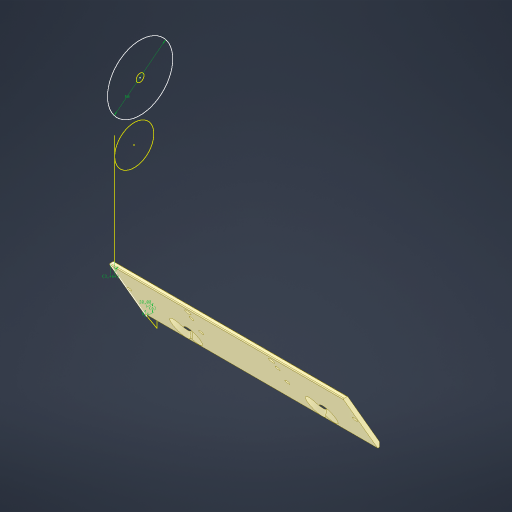
# Autodesk Inventor part: front
Saved by Autodesk Inventor 2023 (Build 270158000, 158)
## iProperties
Created: 2024-05-26
Part Number: front
Material: Nylon 6
Document SubType Name: Modeling
Designer: szymo
Density: 1.12 g/cm^3
Appearance: Nylon 6
Mass: 18.6267 g
Surface Area: 186.523 cm^2
Volume: 16.631 cm^3
TOTAL MASS: 0.0
Author: szymo
Autodesk Inventor part; units mm, degrees
ref_plane "Work Plane1" through (-178, 0.5, -3.5) normal (-1, 0, 0) x (0, 0, 1)
sketch "Sketch1" plane through (-178, 0.5, -3.5) normal (-1, 0, 0) x (0, 0, 1)
  line L0 (3.5, 3.5) -> (-1, 3.5) projected
  line L1 (-1, 3.5) -> (-1, -0.5) projected
  line L2 (-1, -0.5) -> (-4.5, -0.5) projected
  line L3 (-4.5, -0.5) -> (-4.5, -14.5) projected
  line L4 (-4.5, -14.5) -> (4.5, -0.5) projected
  line L5 (4.5, -0.5) -> (3.5, -0.5) projected
  line L6 (3.5, -0.5) -> (3.5, 3.5) projected
  circle A0 centre (8.5, 158.5) radius 3 projected
  circle A1 centre (8.5, 158.5) radius 25
  circle A2 centre (13, 116) radius 15 projected
  line L7 (3.5, 3.5) -> (28, 45.9352)
  line L8 (3.5, -2.5) -> (31.4641, 45.9352)
  line L9 (31.4641, 45.9352) -> (28, 45.9352)
  line L10 (28, 45.9352) -> (28, 130) projected
  line L11 (3.5, -2.5) -> (3.5, -0.5)
  line L12 (3.5, -0.1) -> (4.8856, -0.1)
  point P0 (4.0774, -0.5)
  point P1 (3.5, -2.0556)
  dimension "d0" = 50
  dimension "d1" = 30
  dimension "d3" = 3
  dimension "d4" = 6
  dimension "d5" = 3.4641
  dimension "d49" = 0.4
  constraints: 10 end point, 4 point on line, 2 horizontal, 1 centre point, 1 coincident, 1 parallel, 1 vertical
  measures "d0" diameter of A1
  measures "d1" angle of L7 L6
  measures "d3" distance between parallel lines of L8 L7
  measures "d4" distance of L8.start L0.start
  measures "d5" distance of L7.end L8.end
  measures "d49" distance between parallel lines of L5 L12
ref_plane "Work Plane2" through (0, -14, -8) normal (1, 0, 0) x (0, 1, 0)
extrude "Extrusion1" add sketch "Sketch1" against normal up to surface (178 mm away) contours L7 L9 L8 L12 L6
ref_plane "Work Plane3" through (-141.1151, 26.996, 4.2847) normal (0, -0.9925462, 0.1218693) x (1, 0, 0)
sketch "Sketch3" plane through (-141.1151, 26.996, 4.2847) normal (0, -0.9925462, 0.1218693) x (1, 0, 0)
  line L0 (89.3087, 5.4518) -> (89.3087, -5.4534)
  spline S0 degree 3 poles (89.3087, -5.4534) (89.308, -5.5772) (89.3587, -5.6989) (89.4451, -5.7853) (89.4649, -5.8051) (89.4865, -5.823) (89.5096, -5.8388) (89.529, -5.8521) (89.5494, -5.864) (89.5707, -5.8743) (89.5866, -5.882) (89.603, -5.8889) (89.6197, -5.8948) (89.6699, -5.9125) (89.7231, -5.9218) (89.7769, -5.9215) knots 0 0 0 0 0.5 0.5 0.5 0.614375 0.614375 0.614375 0.710781 0.710781 0.710781 0.783086 0.783086 0.783086 1 1 1 1
  line L1 (89.7769, -5.9215) -> (118.6836, -5.9215)
  spline S1 degree 3 poles (118.6836, -5.9215) (118.8077, -5.9222) (118.9296, -5.8713) (119.1025, -5.6977) (119.1524, -5.5758) (119.1517, -5.4518) knots 0 0 0 0 0.5 0.5 1 1 1 1
  line L2 (119.1517, -5.4518) -> (119.1517, 5.4534)
  spline S2 degree 3 poles (119.1517, 5.4534) (119.1524, 5.5775) (119.1015, 5.6994) (118.9279, 5.8723) (118.806, 5.9222) (118.682, 5.9215) knots 0 0 0 0 0.5 0.5 1 1 1 1
  line L3 (118.682, 5.9215) -> (89.7769, 5.9215)
  spline S3 degree 3 poles (89.7769, 5.9215) (89.6527, 5.9222) (89.5308, 5.8713) (89.3579, 5.6977) (89.308, 5.5758) (89.3087, 5.4518) knots 0 0 0 0 0.5 0.5 1 1 1 1
  circle A0 centre (90.8511, -4.3791) radius 0.5
  circle A1 centre (90.8511, 4.3791) radius 0.5
  circle A2 centre (117.6093, 4.3791) radius 0.5
  circle A3 centre (117.6093, -4.3791) radius 0.5
  arc A4 (104.4919, -1.4512) -> (104.4113, -1.5218) centre (104.5073, -1.55) ccw
  arc A5 (104.4113, 1.5218) -> (104.4113, -1.5218) centre (99.2302, 0) ccw
  arc A6 (104.4113, 1.5218) -> (104.4919, 1.4512) centre (104.5073, 1.55) ccw
  arc A7 (104.4919, 1.4512) -> (104.5716, 1.519) centre (104.4765, 1.55) ccw
  arc A8 (104.5716, -1.519) -> (104.5716, 1.519) centre (109.2302, 0) ccw
  arc A9 (104.5716, -1.519) -> (104.4919, -1.4512) centre (104.4765, -1.55) ccw
  line L4 (-14.6217, 5.4518) -> (-14.6217, -5.4534)
  spline S4 degree 3 poles (-14.6217, -5.4534) (-14.6224, -5.5772) (-14.5717, -5.6989) (-14.4853, -5.7853) (-14.4655, -5.8051) (-14.4439, -5.823) (-14.4208, -5.8388) (-14.4014, -5.8521) (-14.3809, -5.864) (-14.3597, -5.8743) (-14.3438, -5.882) (-14.3274, -5.8889) (-14.3107, -5.8948) (-14.2605, -5.9125) (-14.2073, -5.9218) (-14.1535, -5.9215) knots 0 0 0 0 0.5 0.5 0.5 0.614375 0.614375 0.614375 0.710781 0.710781 0.710781 0.783086 0.783086 0.783086 1 1 1 1
  line L5 (-14.1535, -5.9215) -> (14.7532, -5.9215)
  spline S5 degree 3 poles (14.7532, -5.9215) (14.8773, -5.9222) (14.9992, -5.8713) (15.1721, -5.6977) (15.222, -5.5758) (15.2213, -5.4518) knots 0 0 0 0 0.5 0.5 1 1 1 1
  line L6 (15.2213, -5.4518) -> (15.2213, 5.4534)
  spline S6 degree 3 poles (15.2213, 5.4534) (15.222, 5.5775) (15.1711, 5.6994) (14.9975, 5.8723) (14.8757, 5.9222) (14.7516, 5.9215) knots 0 0 0 0 0.5 0.5 1 1 1 1
  line L7 (14.7516, 5.9215) -> (-14.1535, 5.9215)
  spline S7 degree 3 poles (-14.1535, 5.9215) (-14.2776, 5.9222) (-14.3996, 5.8713) (-14.5725, 5.6977) (-14.6224, 5.5758) (-14.6217, 5.4518) knots 0 0 0 0 0.5 0.5 1 1 1 1
  circle A10 centre (-13.0792, -4.3791) radius 0.5
  circle A11 centre (-13.0792, 4.3791) radius 0.5
  circle A12 centre (13.6789, 4.3791) radius 0.5
  circle A13 centre (13.6789, -4.3791) radius 0.5
  arc A14 (0.5615, -1.4512) -> (0.4809, -1.5218) centre (0.5769, -1.55) ccw
  arc A15 (0.4809, 1.5218) -> (0.4809, -1.5218) centre (-4.7002, 0) ccw
  arc A16 (0.4809, 1.5218) -> (0.5615, 1.4512) centre (0.5769, 1.55) ccw
  arc A17 (0.5615, 1.4512) -> (0.6412, 1.519) centre (0.5461, 1.55) ccw
  arc A18 (0.6412, -1.519) -> (0.6412, 1.519) centre (5.2998, 0) ccw
  arc A19 (0.6412, -1.519) -> (0.5615, -1.4512) centre (0.5461, -1.55) ccw
  circle A20 centre (99.2302, 0) radius 5.4
  circle A21 centre (109.2302, 0) radius 4.9
  circle A22 centre (-4.7002, 0) radius 5.4
  circle A23 centre (5.2998, 0) radius 4.9
  arc A24 (0.5923, 3.0331) -> (0.5923, -3.0331) centre (-4.7002, 0) ccw
  arc A25 (0.5923, -3.0331) -> (0.5923, 3.0331) centre (5.2998, 0) ccw
  arc A26 (104.5227, -3.0331) -> (104.5227, 3.0331) centre (109.2302, 0) ccw
  arc A27 (104.5227, 3.0331) -> (104.5227, -3.0331) centre (99.2302, 0) ccw
  point P0 (141.1151, -7.5427)
  point P1 (104.4877, 1.2324)
  point P2 (104.4113, 1.5218)
  point P3 (104.4113, -1.5218)
  point P4 (104.4877, -1.2324)
  point P5 (104.5716, -1.519)
  point P6 (104.5716, 1.519)
  point P7 (0.5573, 1.2324)
  point P8 (0.4809, 1.5218)
  point P9 (0.4809, -1.5218)
  point P10 (0.5573, -1.2324)
  point P11 (0.6412, -1.519)
  point P12 (0.6412, 1.519)
  dimension "d19" = 0.7
  dimension "d20" = 0.7
  constraints: 8 centre point, 8 point on circle, 4 coincident, 4 concentric, 2 other
  measures "d19" radial gap between concentric circles of A18 A25
  measures "d20" radial gap between concentric circles of A5 A27
extrude "Extrusion2" cut sketch "Sketch3" along normal up to next contours A27 L3 | L3 A27 A26 L1 | L1 A27 | A4 A20 A21 A9 | A5 A20 A21 | A21 A20 A8 | A6 A7 A21 A20 | A21 A20 | A24 L7 | L7 A24 A25 L5 | L5 A24 | A14 A22 A23 A19 | A15 A22 A23 | A23 A22 A18 | A16 A17 A23 A22 | A23 A22
fillet "Fillet1" radius 1 3 edges at (-140.5228, 16.0434, 8.6853) (-140.5228, 7.3141, 3.6455) (-36.5924, 16.0434, 8.6853)
sketch "Sketch4" plane through (-178, 46.4352, 27.9641) normal (0, -0.5, 0.8660254) x (1, 0, 0)
  line L0 (5, -23.2887) -> (5, -26.2887) projected
  line L1 (0, -48.134) -> (0, -1.4434) projected
  line L2 (0, -48.134) -> (3, -48.134) projected
  line L3 (178, -48.134) -> (175, -48.134) projected
  line L4 (178, -48.134) -> (178, -1.4434) projected
  line L5 (173, -23.2887) -> (173, -26.2887) projected
  arc A0 (118.5, -2.2472) -> (117.5, -3.9793) centre (119.5, -3.9793) ccw projected
  line L6 (117.5, -3.9793) -> (117.5, -7.0511) projected
  arc A1 (117.5, -7.0511) -> (118.5, -8.7831) centre (119.5, -7.0511) ccw projected
  arc A2 (119.5, -10.5152) -> (118.5, -8.7831) centre (117.5, -10.5152) ccw projected
  line L7 (119.5, -10.5152) -> (119.5, -33.4952) projected
  line L8 (119.5, -33.4952) -> (124.5, -33.4952) projected
  line L9 (124.5, -1.4434) -> (124.5, -33.4952) projected
  line L10 (124.5, -1.4434) -> (119.2716, -1.4434) projected
  arc A3 (118.5, -2.2472) -> (119.2716, -1.4434) centre (117.5, -0.5152) ccw projected
  circle A4 centre (121, -5.5152) radius 2.3 projected
  circle A5 centre (122, -27.9147) radius 1.75 projected
  circle A6 centre (122, -12.9147) radius 1.75 projected
  arc A7 (60.5, -3.9793) -> (59.5, -2.2472) centre (58.5, -3.9793) ccw projected
  arc A8 (58.7284, -1.4434) -> (59.5, -2.2472) centre (60.5, -0.5152) ccw projected
  line L11 (53.5, -1.4434) -> (58.7284, -1.4434) projected
  line L12 (53.5, -1.4434) -> (53.5, -33.4952) projected
  line L13 (58.5, -33.4952) -> (53.5, -33.4952) projected
  line L14 (58.5, -10.5152) -> (58.5, -33.4952) projected
  arc A9 (59.5, -8.7831) -> (58.5, -10.5152) centre (60.5, -10.5152) ccw projected
  arc A10 (59.5, -8.7831) -> (60.5, -7.0511) centre (58.5, -7.0511) ccw projected
  line L15 (60.5, -3.9793) -> (60.5, -7.0511) projected
  circle A11 centre (57, -5.5152) radius 2.3 projected
  circle A12 centre (56, -27.9147) radius 1.75 projected
  circle A13 centre (56, -12.9147) radius 1.75 projected
  arc A14 (174, -22.2887) -> (173, -23.2887) centre (174, -23.2887) ccw projected
  arc A15 (173, -26.2887) -> (174, -27.2887) centre (174, -26.2887) ccw projected
  arc A16 (175, -28.2887) -> (174, -27.2887) centre (174, -28.2887) ccw projected
  line L16 (175, -28.2887) -> (175, -30.8135) projected
  line L17 (175, -30.8135) -> (175, -48.134) projected
  line L18 (178, -1.4434) -> (174, -1.4434) projected
  ellipse E0 centre (174, -2.5981) end of major axis (174, -1.4434) minor radius 1 (175, -2.5981) -> (174, -1.4434) ccw projected
  line L19 (175, -2.5981) -> (175, -21.2887) projected
  arc A17 (174, -22.2887) -> (175, -21.2887) centre (174, -21.2887) ccw projected
  arc A18 (5, -23.2887) -> (4, -22.2887) centre (4, -23.2887) ccw projected
  arc A19 (3, -21.2887) -> (4, -22.2887) centre (4, -21.2887) ccw projected
  line L20 (3, -2.5981) -> (3, -21.2887) projected
  ellipse E1 centre (4, -2.5981) end of major axis (4, -1.4434) minor radius 1 (4, -1.4434) -> (3, -2.5981) ccw projected
  line L21 (0, -1.4434) -> (4, -1.4434) projected
  line L22 (3, -30.8135) -> (3, -48.134) projected
  line L23 (3, -28.2887) -> (3, -30.8135) projected
  arc A20 (4, -27.2887) -> (3, -28.2887) centre (4, -28.2887) ccw projected
  arc A21 (4, -27.2887) -> (5, -26.2887) centre (4, -26.2887) ccw projected
  circle A22 centre (2.5, -24.7887) radius 1.75 projected
  circle A23 centre (175.5, -24.7887) radius 1.75 projected
  point P0 (178, -54.1962)
  point P1 (2.5, -24.5)
  point P2 (175.5, -24.5)
  point P3 (3, -1.1547)
  point P4 (175, -1.1547)
  constraints: 4 coincident, 4 other
hole "srobkiSrodek" at (-122, 22.2604, 14.0068) at (-122, 35.2508, 21.5068) at (-56, 22.2604, 14.0068) at (-56, 35.2508, 21.5068) direction (0, 0.5, -0.8660254) diameter 3.5 end through all counterbore diameter 6 counterbore depth 0
sketch "Sketch6" plane through (-178, 46.4352, 27.9641) normal (0, -0.5, 0.8660254) x (1, 0, 0)
  circle A0 centre (57, -5.5152) radius 2.3 projected
  circle A1 centre (121, -5.5152) radius 2.3 projected
  point P0 (178, -54.1962)
  constraints: 2 coincident
hole "czulki" at (-57, 41.659, 25.2065) at (-121, 41.659, 25.2065) direction (0, 0.5, -0.8660254) diameter 4.4 end through all
sketch "Sketch7" plane through (-178, 46.4352, 27.9641) normal (0, -0.5, 0.8660254) x (1, 0, 0)
  line L0 (5, -23.2887) -> (5, -26.2887) projected
  line L1 (0, -48.134) -> (0, -1.4434) projected
  line L2 (0, -48.134) -> (3, -48.134) projected
  line L3 (178, -48.134) -> (175, -48.134) projected
  line L4 (178, -48.134) -> (178, -1.4434) projected
  line L5 (173, -23.2887) -> (173, -26.2887) projected
  arc A0 (5, -23.2887) -> (4, -22.2887) centre (4, -23.2887) ccw projected
  arc A1 (3, -21.2887) -> (4, -22.2887) centre (4, -21.2887) ccw projected
  line L6 (3, -2.5981) -> (3, -21.2887) projected
  ellipse E0 centre (4, -2.5981) end of major axis (4, -1.4434) minor radius 1 (4, -1.4434) -> (3, -2.5981) ccw projected
  line L7 (0, -1.4434) -> (4, -1.4434) projected
  line L8 (3, -30.8135) -> (3, -48.134) projected
  line L9 (3, -28.2887) -> (3, -30.8135) projected
  arc A2 (4, -27.2887) -> (3, -28.2887) centre (4, -28.2887) ccw projected
  arc A3 (4, -27.2887) -> (5, -26.2887) centre (4, -26.2887) ccw projected
  circle A4 centre (2.5, -24.7887) radius 1.75 projected
  arc A5 (174, -22.2887) -> (173, -23.2887) centre (174, -23.2887) ccw projected
  arc A6 (173, -26.2887) -> (174, -27.2887) centre (174, -26.2887) ccw projected
  arc A7 (175, -28.2887) -> (174, -27.2887) centre (174, -28.2887) ccw projected
  line L10 (175, -28.2887) -> (175, -30.8135) projected
  line L11 (175, -30.8135) -> (175, -48.134) projected
  line L12 (178, -1.4434) -> (174, -1.4434) projected
  ellipse E1 centre (174, -2.5981) end of major axis (174, -1.4434) minor radius 1 (175, -2.5981) -> (174, -1.4434) ccw projected
  line L13 (175, -2.5981) -> (175, -21.2887) projected
  arc A8 (174, -22.2887) -> (175, -21.2887) centre (174, -21.2887) ccw projected
  circle A9 centre (175.5, -24.7887) radius 1.75 projected
  point P0 (178, -54.1962)
  point P1 (175.5, -24.5)
  point P2 (2.5, -24.5)
  point P3 (175, -1.1547)
  point P4 (3, -1.1547)
  constraints: 4 other
hole "srubkiBoki" at (-2.5, 25.2176, 15.7141) at (-175.5, 25.2176, 15.7141) direction (0, 0.5, -0.8660254) diameter 3.5 end through all
fillet "Fillet2" radius 0.5 5 edges at (-89, 4, 0) (-89, 46.4352, 24.5) (-89, 46.4352, 27.9641) (-89, 0.4, 0) (-89, 0.4, 1.3856)
sketch "Sketch8" plane through (0, 0.9, 0) normal (1, 0, 0) x (0, 0, -1)
  arc A0 (-1.53, -0.25) -> (-1.097, -0.5) centre (-1.097, 0) ccw projected
  line L0 (-0.5, -0.5) -> (-1.097, -0.5) projected
  arc A1 (-0.5, -0.5) -> (0, 0) centre (-0.5, 0) ccw projected
  line L1 (0, 2.966) -> (0, 0) projected
  arc A2 (0, 2.966) -> (-0.067, 3.216) centre (-0.5, 2.966) ccw projected
  line L2 (-24.3557, 45.2852) -> (-0.067, 3.216) projected
  arc A3 (-24.3557, 45.2852) -> (-24.7887, 45.5352) centre (-24.7887, 45.0352) ccw projected
  line L3 (-27.0981, 45.5352) -> (-24.7887, 45.5352) projected
  arc A4 (-27.0981, 45.5352) -> (-27.5311, 44.7852) centre (-27.0981, 45.0352) ccw projected
  line L4 (-1.53, -0.25) -> (-27.5311, 44.7852) projected
  point P0 (0, -0.9)
extrude "Extrusion3" add sketch "Sketch8" along normal blind 0.64
sketch "Sketch9" plane through (-178, 0.5, -3.5) normal (-1, 0, 0) x (0, 0, 1)
  arc A0 (4.597, -0.1) -> (5.03, 0.15) centre (4.597, 0.4) ccw projected
  line L0 (5.03, 0.15) -> (31.0311, 45.1852) projected
  arc A1 (31.0311, 45.1852) -> (30.5981, 45.9352) centre (30.5981, 45.4352) ccw projected
  line L1 (30.5981, 45.9352) -> (28.2887, 45.9352) projected
  arc A2 (28.2887, 45.9352) -> (27.8557, 45.6852) centre (28.2887, 45.4352) ccw projected
  line L2 (27.8557, 45.6852) -> (3.567, 3.616) projected
  arc A3 (3.567, 3.616) -> (3.5, 3.366) centre (4, 3.366) ccw projected
  line L3 (3.5, 3.366) -> (3.5, 0.4) projected
  arc A4 (3.5, 0.4) -> (4, -0.1) centre (4, 0.4) ccw projected
  line L4 (4, -0.1) -> (4.597, -0.1) projected
  point P0 (3.5, -0.5)
extrude "Extrusion4" add sketch "Sketch9" along normal blind 0.75
body "Solid1"
